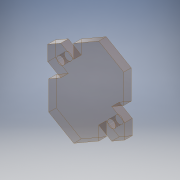
# Autodesk Inventor part: Dribbler Plate
Saved by Autodesk Inventor 2017 (Build 210142000, 142)
## iProperties
Created: 2017-04-14
Part Number: Dribbler Plate
Material: Polycarbonate, Smoke
Document SubType Name: Modeling
Designer: yella
Density: 1.2 g/cm^3
Appearance: Polycarbonate - Smoked
Author: yella
Autodesk Inventor part; units mm, degrees
ref_plane "YZ Plane" through (0, 0, 0) normal (1, 0, 0) x (0, 1, 0)
ref_plane "XZ Plane" through (0, 0, 0) normal (0, 1, 0) x (-1, 0, 0)
ref_plane "XY Plane" through (0, 0, 0) normal (0, 0, 1) x (1, 0, 0)
sketch "Sketch1" plane through (0, 0, 0) normal (0, 1, 0) x (-1, 0, 0)
  line L0 (0, 11.547) -> (10, 5.7735)
  line L1 (10, 5.7735) -> (10, -5.7735)
  line L2 (10, -5.7735) -> (0, -11.547)
  line L3 (0, -11.547) -> (-10, -5.7735)
  line L4 (-10, -5.7735) -> (-10, 5.7735)
  line L5 (-10, 5.7735) -> (0, 11.547)
  line L6 (-10, 5.7735) -> (-20, 11.547)
  line L7 (-20, 11.547) -> (-20, 23.094)
  line L8 (-20, 23.094) -> (-10, 28.8675)
  line L9 (-10, 28.8675) -> (0, 23.094)
  line L10 (0, 23.094) -> (0, 11.547)
  line L11 (0, 11.547) -> (-10, 5.7735)
  circle A0 centre (-15.1962, 2.7735) radius 1.6
  circle A1 centre (5.1962, 14.547) radius 1.6
  line L12 (0, 11.547) -> (5.1962, 14.547)
  line L13 (-10, 5.7735) -> (-15.1962, 2.7735)
  line L14 (-10, 5.7735) -> (-10, -0.2265)
  line L15 (-10, -0.2265) -> (-15.1962, -3.2265)
  line L16 (-15.1962, -3.2265) -> (-20.3923, -0.2265)
  line L17 (-20.3923, -0.2265) -> (-20.3923, 5.7735)
  line L18 (-20.3923, 5.7735) -> (-15.1962, 8.7735)
  line L19 (-15.1962, 8.7735) -> (-10, 5.7735)
  line L20 (0, 11.547) -> (0, 17.547)
  line L21 (0, 17.547) -> (5.1962, 20.547)
  line L22 (5.1962, 20.547) -> (10.3923, 17.547)
  line L23 (10.3923, 17.547) -> (10.3923, 11.547)
  line L24 (10.3923, 11.547) -> (5.1962, 8.547)
  line L25 (5.1962, 8.547) -> (0, 11.547)
  dimension "d26" = 3.2
  dimension "d27" = 3.2
  dimension "d28" = 6
  dimension "d29" = 6
  constraints: 52 end point, 4 coincident, 2 centre point, 26 other
  measures "d26" diameter of A0
  measures "d27" diameter of A1
  measures "d28" distance of L10.end L12.end
  measures "d29" distance of L4.end L13.end
extrude "Extrusion1" add sketch "Sketch1" along normal blind 3
body "Solid1"
